Autodesk Fusion 360 part; units mm, degrees
note: some values were not read from the file. Set by a fixed rule: which sketch regions a step uses.
(part 2 of 2)
extrude "Extrude5" cut sketch "Sketch3" against normal blind 0.5 contours L6 L7 L8 L9 L10 L11 L12 L13 L14 L15 L16 L17 L18 L19 L20 L21 L22 L23 L24 L25 | L26 L27 L28 L29 L30 L31 L32 L33 L34 L35 L36 L37 L38 L39 L40 L41 L42 L43 L44 L45 L46 L47 L48 L49 L50 L51 L52 L53 L54 L55 L56 L57 L58 L59 L60 L61 L62 L63 L64 L65 L66 L67 L68 L69 L70 L71 L72 L73 L74 L75 L76 L77 L78 L79 L80 L81 | L82 L83 L84 L85 L86 L87 L88 L89 L90 L91 L92 L93 L94 L95 L96 L97 L98 L99 L100 L101 L102 L103 L104 L105 | L106 L107 L108 L109 L110 L111 L112 L113 L114 L115 L116 L117 | L118 L119 L120 L121 L122 L123 L124 L125 | L126 L127 L128 L129 L130 L131 L132 L133 L134 L135 L136 L137 L138 L139 L140 L141 L142 L143 | L144 L145 L146 L147 L148 L149 L150 L151 L152 L153 L154 L155 L156 L157 L158 L159 L160 L161 L162 L163 L164 L165 L166 L167 L168 L169 L170 L171 L172 L173 L174 L175 L176 L177 L178 L179 L180 L181 L182 L183 L184 L185 L186 L187 L188 L189 L190 L191 L192 L193 L194 L195 L196 L197 L198 L199 L200 L201 | L202 L203 L204 L205 L206 L207 L208 L209 L210 L211 L212 L213 L214 L215 L216 L217 L218 L219 L220 L221 L222 L223 L224 L225 L226 L227 L228 L229 | L230 L231 L232 L233 L234 L235 L236 L237 L238 L239 L240 L241 | L242 L243 L244 L245 L246 L247 L248 L249 | L250 L251 L252 L253 L254 L255 L256 L257 | L258 L259 L260 L261 L262 L263 L264 L265 | L266 L267 L268 L269 L270 L271 L272 L273 L274 L275 L276 L277 L278 L279 L280 L281 L282 L283 L284 L285 | L286 L287 L288 L289 L290 L291 L292 L293 | L294 L295 L296 L297 L298 L299 L300 L301 L302 L303 L304 L305 L306 L307 L308 L309 L310 L311 L312 L313 | L314 L315 L316 L317 L318 L319 L320 L321 | L322 L323 L324 L325 L326 L327 L328 L329 L330 L331 L332 L333 L334 L335 L336 L337 L338 L339 L340 L341 L342 L343 L344 L345 L346 L347 L348 L349 L350 L351 L352 L353 L354 L355 L356 L357 L358 L359 L360 L361 L362 L363 L364 L365 L366 L367 | L368 L369 L370 L371 L372 L373 L374 L375 L376 L377 L378 L379 L380 L381 L382 L383 L384 L385 L386 L387 L388 L389 L390 L391 | L392 L393 L394 L395 L396 L397 L398 L399 L400 L401 L402 L403 L404 L405 L406 L407 L408 L409 L410 L411 L412 L413 L414 L415 L416 L417 L418 L419 L420 L421 L422 L423 L424 L425 L426 L427 L428 L429 L430 L431 L432 L433 L434 L435 | L436 L437 L438 L439 L440 L441 L442 L443 L444 L445 L446 L447 | L630 L631 L632 L633 L634 L635 L636 L637 L638 L639 L640 L641 L642 L643 L644 L645 L646 L647 L648 L649 L650 L651 L652 L653 L654 L655 L656 L657 L658 L659 L660 L661 L662 L663 L664 L665 L666 L667 L668 L669 L670 L671 L672 L673 L674 L675 L676 L677 L678 L679 | L448 L449 L450 L451 L452 L453 L454 L455 L456 L457 L458 L459 L460 L461 L462 L463 L464 L465 L466 L467 L468 L469 L470 L471 L472 L473 L474 L475 L476 L477 L478 L479 L480 L481 L482 L483 L484 L485 L486 L487 L488 L489 L490 L491 | L492 L493 L494 L495 L496 L497 L498 L499 L500 L501 L502 L503 L504 L505 L506 L507 L508 L509 L510 L511 L512 L513 L514 L515 L516 L517 L518 L519 L520 L521 L522 L523 L524 L525 L526 L527 L528 L529 L530 L531 L532 L533 L534 L535 L536 L537 | L538 L539 L540 L541 L542 L543 L544 L545 L546 L547 L548 L549 L550 L551 L552 L553 L554 L555 L556 L557 L558 L559 L560 L561 | L562 L563 L564 L565 L566 L567 L568 L569 L570 L571 L572 L573 L574 L575 L576 L577 L578 L579 L580 L581 L582 L583 L584 L585 L586 L587 L588 L589 L590 L591 L592 L593 L594 L595 L596 L597 L598 L599 L600 L601 L602 L603 L604 L605 L606 L607 L608 L609 L610 L611 L612 L613 L614 L615 L616 L617 | L618 L619 L620 L621 L622 L623 L624 L625 L626 L627 L628 L629 | L680 L681 L682 L683 L684 L685 L686 L687 L688 L689 L690 L691 | L692 L693 L694 L695 L696 L697 L698 L699
move_face "MoveFace1" by (-0.202, 0, 0) 302 faces at (26.9299, -18.2589, -0.9568) (20.8813, -22.4025, -0.6816) (27.8327, -18.6192, -0.9329) (18.8952, -17.8085, -0.9867) (21.7841, -12.8541, -1.3158) (25.8466, -16.2771, -1.0884) (28.2841, -12.674, -1.3278) (10.9508, -19.52, -0.873) (28.8258, -15.3763, -1.1483) (24.8535, -18.6192, -0.9329) (21.8744, -12.674, -1.3278) (25.2147, -15.6466, -1.1303) (16.9091, -9.6113, -1.5312) (25.0341, -21.1304, -0.599) (15.5549, -15.8267, -1.1183) (16.1869, -15.9058, -0.9461) (25.0341, -15.7367, -1.1243) (16.0966, -14.2843, -1.0538) (23.1383, -17.7184, -0.9927) (14.8327, -15.3763, -1.1483) (13.5688, -18.6192, -0.9329) (29.9091, -15.8267, -1.1183) (7.4299, -18.2589, -0.9568) (22.0549, -12.5728, -1.1674) (27.5619, -17.5382, -1.0047) (19.0758, -17.7184, -0.9927) (29.7285, -18.6192, -0.9329) (21.0619, -18.6192, -0.9329) (21.8744, -11.8632, -1.3816) (9.0549, -18.6192, -0.9329) (21.2424, -21.1304, -0.599) (25.3049, -12.2236, -1.3577) (14.2008, -19.1486, -0.7307) (29.6383, -18.439, -0.9448) (10.6799, -19.7902, -0.8551) (9.5966, -14.7237, -0.8575) (24.673, -22.4025, -0.6816) (28.5549, -16.7275, -1.0585) (21.7841, -16.6374, -1.0645) (8.6938, -9.4311, -1.5431) (10.8605, -19.7001, -0.8611) (22.9577, -17.8085, -0.9867) (14.4716, -12.3136, -1.3517) (12.3049, -18.2589, -0.9568) (29.3674, -11.3228, -1.4175) (16.7285, -9.7013, -1.5252) (26.2077, -15.3763, -1.1483) (16.2772, -13.4736, -1.1076) (10.8605, -10.7823, -1.4534) (26.1174, -20.8712, -0.7833) (22.1452, -18.6192, -0.9329) (28.5549, -9.5212, -1.5372) (24.3119, -9.7013, -1.5252) (22.0584, -16.5244, 1.6665) (28.6452, -9.7013, -1.5252) (15.7856, -18.1608, 1.6665) (23.8605, -11.593, -1.3996) (10.2285, -22.4025, -0.6816) (16.9091, -17.9886, -0.9748) (26.5688, -21.862, -0.7175) (7.9716, -20.0494, -0.6708) (29.2772, -21.862, -0.7175) (22.5966, -11.1426, -1.4295) (11.2216, -21.6819, -0.7294) (15.2841, -20.77, -0.623) (28.3744, -21.0513, -0.7713) (17.541, -17.5382, -1.0047) (7.6105, -21.5918, -0.7354) (16.9994, -17.8085, -0.9867) (23.9508, -12.3136, -1.3517) (10.1383, -20.4097, -0.6469) (23.8605, -12.6629, -1.1615) (18.2633, -17.6283, -0.9987) (7.9716, -21.9411, -0.5452) (28.5549, -20.8601, -0.617) (27.4716, -21.2204, -0.5931) (26.6591, -21.9411, -0.5452) (9.5966, -21.3216, -0.7534) (27.291, -21.0513, -0.7713) (8.1522, -22.1323, -0.6995) (19.7077, -18.8894, -0.9149) (16.0966, -21.1414, -0.7653) (7.4299, -21.2204, -0.5931) (17.1799, -17.7184, -0.9927) (22.5063, -11.3228, -1.4175) (16.8188, -22.4025, -0.6816) (7.791, -20.2406, -0.8252) (18.2633, -20.0605, -0.8371) (29.0966, -21.9521, -0.7115) (9.7772, -20.5109, -0.8072) (18.3535, -17.8085, -0.9867) (23.5897, -11.3228, -1.4175) (17.1799, -21.3105, -0.5871) (22.3258, -11.5029, -1.4055) (8.2424, -22.2113, -0.5273) (29.0063, -22.1323, -0.6995) (29.3674, -21.6819, -0.7294) (23.6799, -11.4919, -1.2392) (7.7008, -20.3196, -0.6529) (28.1938, -22.4025, -0.6816) (23.4091, -11.2327, -1.4235) (28.8258, -22.2224, -0.6936) (23.6799, -12.4938, -1.3397) (28.6452, -20.7811, -0.7893) (14.923, -19.7681, -0.5225) (20.9716, -11.4018, -1.2452) (16.3674, -13.3835, -1.1136) (19.4369, -17.5382, -1.0047) (23.9508, -21.6708, -0.5631) (29.9091, -10.9624, -1.4414) (13.6591, -19.4299, -0.879) (29.6383, -10.6021, -1.4654) (29.7285, -10.7823, -1.4534) (23.6799, -21.3216, -0.7534) (16.6383, -9.8705, -1.3469) (9.8674, -18.9685, -0.7426) (25.1244, -10.5121, -1.4713) (21.423, -16.187, -1.0944) (22.5063, -15.1741, -0.8276) (9.6869, -19.1597, -0.897) (29.3674, -18.1688, -0.9628) (20.9716, -18.439, -0.9448) (29.4577, -18.349, -0.9508) (7.4299, -10.3208, -1.317) (26.9299, -13.3835, -1.1136) (13.298, -17.5382, -1.0047) (22.8674, -17.9886, -0.9748) (15.1938, -10.7823, -1.4534) (28.8258, -9.7914, -1.5192) (24.4924, -9.7914, -1.5192) (16.4577, -20.0384, -0.5045) (28.8258, -20.2296, -0.6589) (22.3258, -18.5291, -0.9389) (21.3327, -13.2144, -1.2919) (16.1869, -10.2418, -1.4893) (16.1869, -12.6629, -1.1615) (9.2355, -17.8765, -0.6481) (11.2216, -9.8815, -1.5132) (21.5133, -13.1244, -1.2978) (28.916, -9.9716, -1.5072) (26.3883, -21.6708, -0.5631) (17.4508, -18.9685, -0.7426) (8.9647, -20.7811, -0.7893) (10.5897, -19.9704, -0.8431) (16.7285, -18.0787, -0.9688) (16.1869, -18.6192, -0.9329) (17.9924, -19.0585, -0.7367) (9.0549, -20.5899, -0.6349) (28.2841, -21.1304, -0.599) (26.9299, -22.2113, -0.5273) (18.173, -19.1597, -0.897) (7.8813, -21.862, -0.7175) (7.7008, -21.6708, -0.5631) (27.2008, -20.8712, -0.7833) (16.6383, -18.2589, -0.9568) (17.3605, -19.1597, -0.897) (7.5202, -20.5109, -0.8072) (27.0202, -20.7811, -0.7893) (26.9299, -20.5899, -0.6349) (27.6522, -20.5109, -0.8072) (27.7424, -21.3216, -0.7534) (10.3188, -20.2406, -0.8252) (17.8119, -18.8894, -0.9149) (16.4577, -18.349, -0.9508) (10.4091, -20.0605, -0.8371) (8.7841, -20.9612, -0.7773) (26.8397, -22.1323, -0.6995) (8.0619, -19.9704, -0.8431) (16.3674, -18.5291, -0.9389) (26.298, -21.5918, -0.7354) (16.4577, -13.2144, -1.2919) (13.3883, -20.1505, -0.8312) (21.5133, -16.3672, -1.0824) (16.4577, -9.9716, -1.5072) (29.1869, -18.0787, -0.9688) (20.791, -18.349, -0.9508) (8.1522, -10.7823, -1.4534) (21.2424, -16.097, -1.1004) (29.4577, -10.5121, -1.4713) (22.6869, -18.0787, -0.9688) (22.7772, -9.4311, -1.5431) (9.5966, -19.3398, -0.885) (29.0966, -17.8986, -0.9807) (8.8744, -19.4299, -0.879) (28.916, -17.8085, -0.9867) (8.2424, -19.8803, -0.8491) (16.6383, -13.1244, -1.2978) (27.3813, -12.0213, -1.037) (13.9299, -20.5109, -0.8072) (15.5549, -9.8815, -1.5132) (20.7008, -18.1688, -0.9628) (21.0619, -15.9058, -0.9461) (23.1383, -21.6819, -0.7294) (25.0341, -10.3319, -1.4833) (8.3327, -19.7001, -0.8611) (29.3674, -10.3319, -1.4833) (14.2008, -21.0403, -0.605) (10.1383, -12.764, -1.3218) (22.5966, -18.2589, -0.9568) (20.4299, -17.8986, -0.9807) (24.8535, -10.2418, -1.4893) (20.5202, -18.0787, -0.9688) (16.3674, -10.1517, -1.4953) (21.6938, -16.4573, -1.0765) (27.4716, -9.4311, -1.5431) (28.8258, -17.6283, -0.9987) (8.5133, -14.7458, -1.1901) (21.2424, -13.3835, -1.1136) (16.4577, -12.9331, -1.1435) (20.2494, -17.8085, -0.9867) (29.1869, -10.2418, -1.4893) (22.7772, -22.4025, -0.6816) (24.7633, -10.0617, -1.5013) (12.9369, -21.3216, -0.7534) (20.9716, -14.2843, -1.0538) (16.3674, -12.8541, -1.3158) (8.5133, -19.6101, -0.8671) (29.548, -20.2185, -0.4926) (18.8049, -17.9886, -0.9748) (11.2216, -18.6982, -0.7606) (18.5341, -17.8986, -0.9807) (28.2841, -18.7993, -0.9209) (20.1591, -21.3216, -0.7534) (11.1313, -19.4299, -0.879) (23.6799, -19.4979, -0.5404) (24.8535, -15.9058, -0.9461) (8.423, -17.5382, -1.0047) (21.0619, -10.5121, -1.4713) (24.673, -16.187, -1.0944) (18.4438, -13.0122, -0.9712) (21.2424, -10.422, -1.4773) (17.7216, -9.4311, -1.5431) (11.7633, -16.2771, -1.0884) (16.3674, -16.097, -1.1004) (24.7633, -18.439, -0.9448) (28.4647, -18.8894, -0.9149) (23.4091, -17.5382, -1.0047) (14.291, -16.7275, -1.0585) (24.7633, -16.0069, -1.1064) (21.6938, -12.9331, -1.1435) (28.5549, -19.0585, -0.7367) (13.0272, -9.4311, -1.5431) (19.2563, -19.1597, -0.897) (24.041, -17.8085, -0.9867) (21.8744, -9.7013, -1.5252) (24.2216, -16.5474, -1.0705) (10.4091, -17.6283, -0.9987) (11.041, -18.349, -0.9508) (29.548, -21.5918, -0.7354) (13.9299, -13.8229, -0.9174) (26.7494, -19.4299, -0.879) (18.5341, -16.7275, -1.0585) (10.6799, -17.8986, -0.9807) (18.8049, -20.5109, -0.8072) (10.5897, -17.7974, -0.8204) (24.2216, -17.8986, -0.9807) (23.4091, -16.7275, -1.0585) (24.5827, -18.349, -0.9508) (16.548, -16.187, -1.0944) (24.4022, -16.4573, -1.0765) (21.5133, -10.1517, -1.4953) (19.3466, -14.2843, -1.0538) (22.0549, -9.6113, -1.5312) (19.3466, -18.9685, -0.7426) (29.8188, -21.3216, -0.7534) (10.7702, -18.0787, -0.9688) (19.0758, -20.0494, -0.6708) (16.9091, -16.6374, -1.0645) (21.3327, -10.2418, -1.4893) (24.4924, -16.2771, -1.0884) (11.7633, -10.3208, -1.317) (16.8188, -16.4573, -1.0765) (19.8883, -19.0585, -0.7367) (10.9508, -18.1688, -0.9628) (24.3119, -18.0787, -0.9688) (23.9508, -17.6283, -0.9987) (29.6383, -21.4116, -0.7474) (12.4855, -10.7823, -1.4534) (20.0688, -19.1597, -0.897) (16.6383, -16.3672, -1.0824) (12.1244, -15.3763, -1.1483) (18.6244, -18.0787, -0.9688) (24.4924, -18.1688, -0.9628) (28.0133, -19.7902, -0.8551) (12.8466, -13.8339, -1.0837) (28.7355, -19.1597, -0.897) (22.5966, -12.4037, -1.3457) (21.6035, -9.9716, -1.5072) (21.7841, -9.8705, -1.3469) (23.1383, -11.0525, -1.4354) (22.0549, -21.1414, -0.7653) (29.0966, -10.0617, -1.5013) (29.9091, -20.4208, -0.8132) (24.5827, -9.9716, -1.5072) (16.0966, -11.8522, -1.2153) (9.5966, -16.7275, -1.0585) (12.3049, -21.6708, -0.5631) (21.1522, -13.4736, -1.1076) (22.416, -18.349, -0.9508) (14.291, -22.4025, -0.6816) (24.2216, -9.5212, -1.5372) (20.1591, -17.6283, -0.9987)
equation "d5 = 39 / 37.835"
equation "d8 = 1.546 mm - 0.5 mm"
named bodies: "Key Chain - 2DS"
